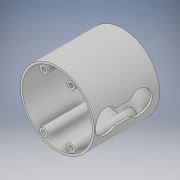
# Autodesk Inventor part: LidarLiteV3Lid
Saved by Autodesk Inventor 2019 (Build 230136000, 136)
## iProperties
Created: 2018-05-28
Part Number: LidarLiteV3Lid
Material: Generic
Document SubType Name: Modeling
Designer: samps
Density: 1 g/cm^3
Appearance: Default
Author: samps
Autodesk Inventor part; units mm, degrees
ref_plane "YZ Plane" through (0, 0, 0) normal (1, 0, 0) x (0, 1, 0)
ref_plane "XZ Plane" through (0, 0, 0) normal (0, 1, 0) x (-1, 0, 0)
ref_plane "XY Plane" through (0, 0, 0) normal (0, 0, 1) x (1, 0, 0)
sketch "Sketch1" plane through (0, 0, 0) normal (0, 0, 1) x (1, 0, 0)
  circle A0 centre (0, 0) radius 31.206
  dimension "d0" = 62.412
  constraints: 1 centre point, 1 coincident
  measures "d0" diameter of A0
extrude "Extrusion1" add sketch "Sketch1" along normal blind 3.175
sketch "Sketch2" plane through (0, 0, 3.175) normal (0, 0, 1) x (1, 0, 0)
  circle A0 centre (0, 0) radius 31.206
  circle A1 centre (0, 0) radius 29.5
  dimension "d3" = 59
  constraints: 2 centre point, 2 coincident
  measures "d3" diameter of A1
sketch "Sketch3" plane through (0, 0, 3.175) normal (0, 0, 1) x (1, 0, 0)
  line L0 (0, 0) -> (-20, 0)
  line L1 (-20, 0) -> (-20, 18)
  line L2 (-20, 18) -> (-23.175, 18)
  line L3 (-23.175, 18) -> (-23.175, -18)
  line L4 (-23.175, -18) -> (-20, -18)
  line L5 (-20, -18) -> (-20, 18)
  dimension "d4" = 20
  dimension "d5" = 18
  dimension "d6" = 3.175
  dimension "d7" = 36
  constraints: 12 end point, 2 horizontal, 2 parallel, 1 perpendicular, 1 vertical
  measures "d4" distance of L0.start L0.end
  measures "d5" distance of L0.end L1.end
  measures "d6" distance of L4.end L3.end
  measures "d7" distance of L3.end L2.end
extrude "Extrusion2" add sketch "Sketch3" along normal blind 52
sketch "Sketch4" plane through (-20, -18, 3.175) normal (1, 0, 0) x (0, 0, -1)
  line L0 (0, 49.206) -> (0, -13.206) projected
  line L1 (-52, 36) -> (-52, 0) projected
  line L2 (-27, 18) -> (-3, 18)
  line L3 (-3, 18) -> (-51, 18)
  line L4 (-27, 18) -> (-41, 18)
  line L5 (-41, 18) -> (-13, 18)
  circle A0 centre (-41, 18) radius 10
  circle A1 centre (-13, 18) radius 10
  line L6 (-13, 18) -> (-41, 18)
  line L7 (-41, 18) -> (-41, 24.5)
  line L8 (-41, 24.5) -> (-13, 24.5)
  line L9 (-13, 24.5) -> (-13, 18)
  line L10 (-41, 24.5) -> (-13, 24.5)
  line L11 (-13, 24.5) -> (-13, 11.5)
  line L12 (-13, 11.5) -> (-41, 11.5)
  line L13 (-41, 11.5) -> (-41, 24.5)
  point P0 (3.175, 18)
  dimension "d34" = 24
  dimension "d35" = 48
  dimension "d36" = 14
  dimension "d37" = 28
  dimension "d38" = 20
  dimension "d39" = 20
  dimension "d40" = 6.5
  dimension "d41" = 13
  constraints: 24 end point, 4 parallel, 3 point on line, 2 centre point, 2 coincident, 2 horizontal, 2 perpendicular
  measures "d34" distance of L2.start L2.end
  measures "d35" distance of L2.end L3.end
  measures "d36" distance of L2.start L4.end
  measures "d37" distance of L4.end L5.end
  measures "d38" diameter of A0
  measures "d39" diameter of A1
  measures "d40" distance of L6.end L7.end
  measures "d41" distance of L10.end L11.end
extrude "Extrusion3" add sketch "Sketch2" along normal blind 52
sketch "Sketch5" plane through (0, 0, 3.175) normal (0, 0, 1) x (1, 0, 0)
  line L0 (0, 0) -> (0, 23)
  line L1 (0, 23) -> (11.5, 23)
  line L2 (11.5, 23) -> (-11.5, 23)
  line L3 (-11.5, 23) -> (-11.5, -23)
  line L4 (-11.5, -23) -> (11.5, -23)
  line L5 (11.5, -23) -> (11.5, 23)
  circle A0 centre (-11.5, 23) radius 3.5
  circle A1 centre (11.5, 23) radius 3.5
  circle A2 centre (-11.5, -23) radius 3.5
  circle A3 centre (11.5, -23) radius 3.5
  dimension "d16" = 23
  dimension "d17" = 11.5
  dimension "d18" = 23
  dimension "d19" = 46
  dimension "d20" = 7
  dimension "d21" = 7
  dimension "d22" = 7
  dimension "d23" = 7
  constraints: 12 end point, 4 centre point, 4 coincident, 2 parallel, 2 perpendicular, 1 horizontal, 1 vertical
  measures "d16" distance of L0.start L0.end
  measures "d17" distance of L0.end L1.end
  measures "d18" distance of L4.end L3.end
  measures "d19" distance of L3.end L2.end
  measures "d20" diameter of A0
  measures "d21" diameter of A1
  measures "d22" diameter of A2
  measures "d23" diameter of A3
extrude "Extrusion4" add sketch "Sketch5" along normal blind 52 contours A1 L5 L1 | L1 L5 A1 | A0 L3 L2 | L2 L3 A0 | A3 L4 L5 | L5 L4 A3 | A2 L4 L3 | L3 L4 A2
sketch "Sketch6" plane through (-11.5, 23, 55.175) normal (0, 0, 1) x (1, 0, 0)
  circle A0 centre (0, 0) radius 3.5 projected
  circle A1 centre (23, 0) radius 3.5 projected
  circle A2 centre (23, -46) radius 3.5 projected
  circle A3 centre (0, -46) radius 3.5 projected
  point P0 (11.5, -23)
  constraints: 4 coincident
hole "Hole1" at (-11.5, 23, 55.175) at (11.5, 23, 55.175) at (11.5, -23, 55.175) at (-11.5, -23, 55.175) direction (0, 0, -1) diameter 3.5 depth 3.5
extrude "Extrusion5" cut sketch "Sketch4" along normal blind 52
sketch "Sketch7" plane through (0, 0, 55.175) normal (0, 0, 1) x (1, 0, 0)
  line L0 (-20, 18) -> (-23.175, 18) projected
  line L1 (-23.175, 18) -> (-23.175, -18) projected
  line L2 (-20, 18) -> (-23.175, 18)
  line L3 (-23.175, 18) -> (-23.175, -18)
  line L4 (-23.175, -18) -> (-20, -18)
  line L5 (-20, -18) -> (-20, 18)
  point P0 (0, 0)
  constraints: 8 end point, 2 parallel, 1 horizontal, 1 perpendicular
extrude "Extrusion6" cut sketch "Sketch7" against normal blind 52
body "Solid1"
